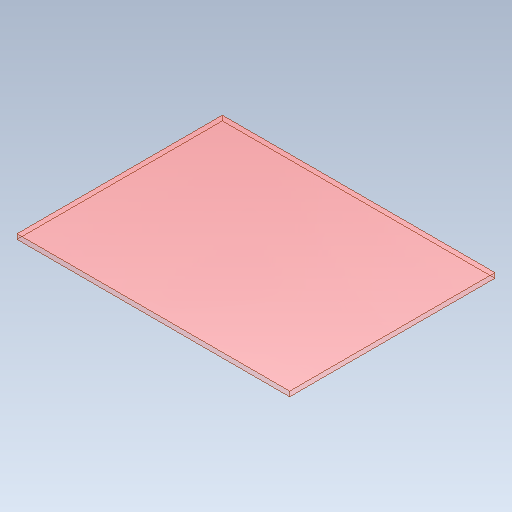
# Autodesk Inventor part: Device Chiplet
Saved by Autodesk Inventor 2021 (Build 250183000, 183)
## iProperties
Created: 2020-04-23
Part Number: Device Chiplet
Material: Polycarbonate, Smoke
Document SubType Name: Modeling
Designer: jgray
Density: 1.2 g/cm^3
Appearance: Polycarbonate - Smoked
Author: jgray
Autodesk Inventor part; units mm, degrees
ref_plane "YZ Plane" through (0, 0, 0) normal (1, 0, 0) x (0, 1, 0)
ref_plane "XZ Plane" through (0, 0, 0) normal (0, 1, 0) x (-1, 0, 0)
ref_plane "XY Plane" through (0, 0, 0) normal (0, 0, 1) x (1, 0, 0)
sketch "Sketch1" plane through (0, 0, 0) normal (0, 1, 0) x (-1, 0, 0)
  line L0 (8.3, 6.25) -> (-8.3, 6.25)
  line L1 (-8.3, 6.25) -> (-8.3, -6.25)
  line L2 (-8.3, -6.25) -> (8.3, -6.25)
  line L3 (8.3, -6.25) -> (8.3, 6.25)
  line L4 (8.3, 6.25) -> (-8.3, -6.25) construction
  line L5 (-8.3, 6.25) -> (8.3, -6.25) construction
  point P0 (0, 0)
  dimension "d0" = 16.6
  dimension "d1" = 12.5
  constraints: 12 end point, 2 midpoint, 2 parallel, 1 horizontal, 1 perpendicular
  measures "d0" distance of L2.end L1.end
  measures "d1" distance of L1.end L0.end
extrude "Extrusion1" add sketch "Sketch1" along normal blind 0.3
body "Solid1"
